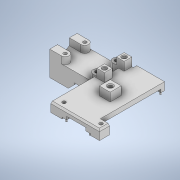
# Autodesk Inventor part: IMU_Mount
Saved by Autodesk Inventor 2022 (Build 260153000, 153)
## iProperties
Created: 2021-10-21
Part Number: IMU_Mount
Material: Generic
Document SubType Name: Modeling
Designer: kylem
Density: 1 g/cm^3
Appearance: Default
Author: kylem
Autodesk Inventor part; units mm, degrees
ref_plane "YZ Plane" through (0, 0, 0) normal (1, 0, 0) x (0, 1, 0)
ref_plane "XZ Plane" through (0, 0, 0) normal (0, 1, 0) x (-1, 0, 0)
ref_plane "XY Plane" through (0, 0, 0) normal (0, 0, 1) x (1, 0, 0)
sketch "Sketch1" plane through (0, 0, 0) normal (0, 1, 0) x (-1, 0, 0)
  point P0 (0, 0)
sketch "Sketch2" plane through (0, 0, 0) normal (0, 1, 0) x (-1, 0, 0)
  line L0 (0, 0) -> (25.5, 0)
  line L1 (25.5, 0) -> (25.5, -17.7)
  line L2 (25.5, -17.7) -> (0, -17.7)
  line L3 (0, -17.7) -> (0, 0)
  line L4 (0, 0) -> (2.5, 0)
  line L5 (2.5, 0) -> (2.5, -2.5)
  line L6 (2.5, -2.5) -> (0, -2.5)
  line L7 (0, -2.5) -> (0, 0)
  circle A0 centre (2.5, -2.5) radius 1
  line L8 (12.75, 0) -> (12.75, -1.25)
  line L9 (0, -8.85) -> (1.25, -8.85)
  circle A1 centre (2.5, -15.2) radius 1
  circle A2 centre (23, -2.5) radius 1
  circle A3 centre (23, -15.2) radius 1
  dimension "d0" = 25.5
  dimension "d1" = 17.7
  dimension "d2" = 2.5
  dimension "d3" = 2.5
  dimension "d4" = 2
  constraints: 20 end point, 4 centre point, 4 parallel, 3 horizontal, 3 symmetric about line, 2 midpoint, 2 perpendicular, 1 coincident, 1 vertical, 3 other
  measures "d0" distance of L1.end L2.end
  measures "d1" distance of L0.end L1.end
  measures "d2" distance of L5.end L6.end
  measures "d3" distance of L4.end L5.end
  measures "d4" diameter of A0
extrude "Extrusion1" add sketch "Sketch2" along normal blind 3 contours L0 L5 A0 L6 L3 | L0 L1 L2 L3 L6 A0 L5
sketch "Sketch3" plane through (0, 3, 0) normal (0, 1, 0) x (1, 0, 0)
  circle A0 centre (-2.5, 2.5) radius 1 projected
  circle A1 centre (-2.5, 2.5) radius 2.5
  circle A2 centre (-23, 2.5) radius 1 projected
  circle A3 centre (-23, 2.5) radius 2.5
  circle A4 centre (-23, 15.2) radius 1 projected
  circle A5 centre (-23, 15.2) radius 2.5
  circle A6 centre (-2.5, 15.2) radius 1 projected
  circle A7 centre (-2.5, 15.2) radius 2.5
  point P0 (0, 0)
  dimension "d7" = 5
  dimension "d8" = 5
  dimension "d9" = 5
  dimension "d10" = 5
  constraints: 4 centre point, 4 coincident
  measures "d7" diameter of A1
  measures "d8" diameter of A3
  measures "d9" diameter of A5
  measures "d10" diameter of A7
extrude "Extrusion2" add sketch "Sketch3" along normal blind 3.5
sketch "Sketch5" plane through (-2.5, 6.5, -15.2) normal (0, 1, 0) x (1, 0, 0)
  line L0 (0, 0) -> (0, 2.5)
  line L1 (2.5, 2.5) -> (-23, 2.5) projected
  line L2 (0, 2.5) -> (35, 2.5)
  line L3 (35, 2.5) -> (35, -15.2)
  line L4 (35, -15.2) -> (0, -15.2)
  line L5 (0, -15.2) -> (0, 2.5)
  circle A0 centre (0, 0) radius 1
  circle A1 centre (0, -12.7) radius 1 projected
  circle A2 centre (0, -12.7) radius 1
  point P0 (2.5, -15.2)
  point P1 (0, 1)
  point P2 (0, -1)
  point P3 (0, -11.7)
  point P4 (0, -13.7)
  dimension "d13" = 35
  constraints: 10 end point, 2 centre point, 2 coincident, 2 parallel, 1 horizontal, 1 perpendicular, 1 point on line, 1 vertical
  measures "d13" distance of L3.end L4.end
extrude "Extrusion3" add sketch "Sketch5" against normal blind 6.5 contours L0 L1 L2 L3 L4 L5 A1 A0
sketch "Sketch6" plane through (0, 6.5, 0) normal (0, 1, 0) x (1, 0, 0)
  line L0 (-2.5, 5) -> (-2.5, 12.7) projected
  line L1 (-2.5, 5) -> (1.5, 5)
  line L2 (1.5, 5) -> (1.5, 12.7)
  line L3 (1.5, 12.7) -> (-2.5, 12.7)
  line L4 (-2.5, 12.7) -> (-2.5, 5)
  point P0 (0, 0)
  dimension "d16" = 4
  constraints: 8 end point, 2 parallel, 1 horizontal, 1 perpendicular
  measures "d16" distance of L3.end L2.end
extrude "Extrusion4" cut sketch "Sketch6" against normal blind 3.5
sketch "Sketch7" plane through (0, 0, 0) normal (0, -1, 0) x (1, 0, 0)
  line L0 (0, 0) -> (4, 0)
  line L1 (-25.5, 0) -> (32.5, 0) projected
  line L2 (4, 0) -> (4, -17.7)
  line L3 (32.5, -17.7) -> (-25.5, -17.7) projected
  line L4 (4, -17.7) -> (32.5, -17.7)
  line L5 (32.5, -17.7) -> (32.5, 0)
  line L6 (32.5, 0) -> (4, 0)
  line L7 (4, 0) -> (4, -17.7)
  dimension "d19" = 4
  constraints: 12 end point, 2 parallel, 2 perpendicular, 2 point on line, 1 horizontal
  measures "d19" distance of L0.start L0.end
extrude "Extrusion5" cut sketch "Sketch7" against normal blind 3.5
sketch "Sketch9" plane through (0, 0, 0) normal (0, -1, 0) x (1, 0, 0)
  circle A0 centre (-23, -2.5) radius 1 projected
  circle A1 centre (-23, -2.5) radius 1
  circle A2 centre (-23, -15.2) radius 2.5 projected
  circle A3 centre (-23, -15.2) radius 1
  arc A4 (-23, 0) -> (-25.5, -2.5) centre (-23, -2.5) ccw projected
  line L0 (-23, 0) -> (-31, 0)
  line L1 (-31, 0) -> (-31, -17.7)
  line L2 (-31, -17.7) -> (-23, -17.7)
  line L3 (-23, -17.7) -> (-23, 0)
  circle A5 centre (-23, -15.2) radius 1
  point P0 (0, 0)
  point P1 (-23, -12.7)
  point P2 (-23, -3.5)
  point P3 (-23, -1.5)
  point P4 (-23, -14.2)
  point P5 (-23, -16.2)
  dimension "d22" = 8
  constraints: 8 end point, 3 centre point, 3 coincident, 2 parallel, 1 horizontal, 1 perpendicular
  measures "d22" distance of L2.end L1.end
extrude "Extrusion6" add sketch "Sketch9" against normal blind 6.5
sketch "Sketch12" plane through (0, 6.5, 0) normal (0, 1, 0) x (1, 0, 0)
  line L0 (-23, 17.7) -> (-31, 17.7) projected
  line L1 (-31, 17.7) -> (-26, 17.7)
  line L2 (-26, 17.7) -> (-26, 12.7)
  line L3 (-26, 12.7) -> (-31, 12.7)
  line L4 (-31, 12.7) -> (-31, 17.7)
  line L5 (-31, 17.7) -> (-31, 0) projected
  line L6 (-31, 0) -> (-26, 0)
  line L7 (-26, 0) -> (-26, 5)
  line L8 (-26, 5) -> (-31, 5)
  line L9 (-31, 5) -> (-31, 0)
  point P0 (0, 0)
  point P1 (-31, 5)
  point P2 (-26, 17.7)
  dimension "d36" = 5
  dimension "d37" = 5
  dimension "d38" = 5
  dimension "d39" = 5
  constraints: 16 end point, 4 parallel, 2 horizontal, 2 perpendicular
  measures "d36" distance of L2.end L3.end
  measures "d37" distance of L1.end L2.end
  measures "d38" distance of L8.end L7.end
  measures "d39" distance of L7.end L6.end
extrude "Extrusion9" add sketch "Sketch12" along normal blind 5.5
sketch "Sketch13" plane through (0, 12, 0) normal (0, 1, 0) x (1, 0, 0)
  line L0 (-26, 17.7) -> (-26, 12.7) projected
  line L1 (-26, 15.2) -> (-28, 15.2)
  line L2 (-31, 0) -> (-31, 17.7) projected
  circle A0 centre (-28, 15.2) radius 1.375
  line L3 (-26, 5) -> (-26, 0) projected
  line L4 (-26, 2.5) -> (-28, 2.5)
  circle A1 centre (-28, 2.5) radius 1.375
  point P0 (0, 0)
  dimension "d42" = 2
  dimension "d43" = 2.75
  dimension "d44" = 2
  dimension "d45" = 2.75
  constraints: 4 end point, 2 centre point, 2 coincident, 2 midpoint, 1 horizontal, 1 perpendicular
  measures "d42" distance of L1.start L1.end
  measures "d43" diameter of A0
  measures "d44" distance of L4.start L4.end
  measures "d45" diameter of A1
extrude "Extrusion10" cut sketch "Sketch13" against normal blind 20
sketch "Sketch14" plane through (4, 0, 0) normal (1, 0, 0) x (0, 0, -1)
  line L0 (0, 0) -> (0, 3.5) projected
  line L1 (17.7, 3.5) -> (0, 3.5) projected
  line L2 (0, 0) -> (17.7, 0)
  line L3 (17.7, 0) -> (17.7, 3.5)
  line L4 (17.7, 3.5) -> (0, 3.5)
  line L5 (0, 3.5) -> (0, 0)
  constraints: 8 end point, 2 parallel, 1 horizontal, 1 perpendicular
extrude "Extrusion11" add sketch "Sketch14" along normal blind 2
sketch "Sketch15" plane through (0, 0, 0) normal (0, -1, 0) x (1, 0, 0)
  line L0 (6, 0) -> (6, -17.7) projected
  line L1 (6, 0) -> (2.5, 0)
  line L2 (2.5, 0) -> (2.5, -2.5)
  line L3 (2.5, -2.5) -> (6, -2.5)
  line L4 (6, -2.5) -> (6, 0)
  line L5 (6, -17.7) -> (2.5, -17.7)
  line L6 (2.5, -17.7) -> (2.5, -15.2)
  line L7 (2.5, -15.2) -> (6, -15.2)
  line L8 (6, -15.2) -> (6, -17.7)
  circle A0 centre (2.5, -2.5) radius 1.375
  circle A1 centre (2.5, -15.2) radius 1.375
  point P0 (0, 0)
  dimension "d50" = 3.5
  dimension "d51" = 2.5
  dimension "d52" = 3.5
  dimension "d53" = 2.5
  dimension "d54" = 2.75
  dimension "d55" = 2.75
  constraints: 16 end point, 4 parallel, 2 centre point, 2 coincident, 2 horizontal, 2 perpendicular
  measures "d50" distance of L3.end L2.end
  measures "d51" distance of L2.end L1.end
  measures "d52" distance of L6.end L7.end
  measures "d53" distance of L5.end L6.end
  measures "d54" diameter of A0
  measures "d55" diameter of A1
extrude "Extrusion12" cut sketch "Sketch15" against normal blind 19 contours A0 L2 L3 | L3 L2 A0 | A1 L6 L7 | L7 L6 A1
sketch "Sketch16" plane through (0, 6.5, 0) normal (0, 1, 0) x (1, 0, 0)
  arc A0 (-23, 12.7) -> (-23, 17.7) centre (-23, 15.2) ccw projected
  circle A1 centre (-23, 15.2) radius 1
  arc A2 (-23, 0) -> (-23, 5) centre (-23, 2.5) ccw projected
  circle A3 centre (-23, 2.5) radius 1
  point P0 (0, 0)
  dimension "d58" = 2
  dimension "d59" = 2
  constraints: 2 centre point, 2 coincident
  measures "d58" diameter of A1
  measures "d59" diameter of A3
extrude "Extrusion13" cut sketch "Sketch16" against normal blind 19
sketch "Sketch18" plane through (0, 3.5, 0) normal (0, -1, 0) x (1, 0, 0)
  line L0 (6, 0) -> (6, -17.7) projected
  line L1 (6, 0) -> (16, 0)
  line L2 (16, 0) -> (16, -5)
  line L3 (16, -5) -> (6, -5)
  line L4 (6, -5) -> (6, 0)
  line L5 (32.5, 0) -> (32.5, -17.7) projected
  line L6 (32.5, -17.7) -> (6, -17.7)
  line L7 (6, -17.7) -> (6, 0)
  line L8 (6, 0) -> (32.5, 0)
  line L9 (32.5, 0) -> (32.5, -17.7)
  point P0 (0, 0)
  point P1 (6, -17.7)
  point P2 (6, -5)
  dimension "d66" = 10
  dimension "d67" = 5
  constraints: 16 end point, 4 parallel, 2 horizontal, 2 perpendicular
  measures "d66" distance of L2.end L3.end
  measures "d67" distance of L1.end L2.end
extrude "Extrusion15" cut sketch "Sketch18" against normal blind 19 contours L3 L2 L8 L5 L6 L0
sketch "Sketch19" plane through (0, 6.5, 0) normal (0, 1, 0) x (1, 0, 0)
  line L0 (6, 0) -> (6, 17.7) projected
  line L1 (-2.5, 0) -> (16, 0) projected
  line L2 (6, 4.9914) -> (16, 4.9914)
  line L3 (16, 4.9914) -> (16, 0)
  line L4 (16, 0) -> (6, 0)
  line L5 (6, 0) -> (6, 4.9914)
  line L6 (6, 0) -> (16, 0)
  line L7 (16, 0) -> (16, -16)
  line L8 (16, -16) -> (6, -16)
  line L9 (6, -16) -> (6, 0)
  line L10 (16, -16) -> (28.75, -16)
  line L11 (28.75, -16) -> (28.75, -24)
  line L12 (28.75, -24) -> (16, -24)
  line L13 (16, -24) -> (16, -16)
  line L14 (16, -24) -> (6, -24)
  line L15 (6, -24) -> (6, -16)
  line L16 (6, -16) -> (16, -16)
  line L17 (16, -16) -> (16, -24)
  point P0 (0, 0)
  point P1 (6, 0)
  dimension "d70" = 16
  dimension "d71" = 12.75
  dimension "d72" = 8
  constraints: 32 end point, 8 parallel, 4 horizontal, 4 perpendicular, 2 point on line
  measures "d70" distance of L6.end L7.end
  measures "d71" distance of L11.end L12.end
  measures "d72" distance of L10.end L11.end
extrude "Extrusion16" add sketch "Sketch19" against normal blind 3 contours L1 L7 L8 L9 | L8 L13 L14 L15 | L10 L11 L12 L13
sketch "Sketch20" plane through (6, 6.5, 0) normal (-1, 0, 0) x (0, 0, 1)
  line L0 (24, 0) -> (16, 0) projected
  line L1 (0, -3) -> (0, -6.5) projected
  line L2 (24, 0) -> (0, 0)
  line L3 (0, 0) -> (0, -3)
  line L4 (0, -3) -> (24, -3)
  line L5 (24, -3) -> (24, 0)
  point P0 (16, 0)
  constraints: 8 end point, 2 parallel, 1 horizontal, 1 perpendicular
extrude "Extrusion17" add sketch "Sketch20" along normal blind 7.5
sketch "Sketch21" plane through (-31, 0, -17.7) normal (-1, 0, 0) x (0, 0, 1)
  line L0 (17.7, 12) -> (12.7, 12) projected
  line L1 (0, 0) -> (17.7, 0)
  line L2 (17.7, 0) -> (17.7, 12)
  line L3 (17.7, 12) -> (0, 12)
  line L4 (0, 12) -> (0, 0)
  point P0 (17.7, 0)
  constraints: 8 end point, 2 parallel, 1 horizontal, 1 perpendicular
extrude "Extrusion18" cut sketch "Sketch21" against normal blind 1
sketch "Sketch22" plane through (0, 6.5, 0) normal (0, 1, 0) x (1, 0, 0)
  circle A0 centre (2.5, 2.5) radius 1.375 projected
  line L0 (2.5, 2.5) -> (0.5, 2.5)
  line L1 (0.5, 2.5) -> (0.5, 0)
  line L2 (0.5, 0) -> (4.5, 0)
  line L3 (4.5, 0) -> (4.5, 5)
  line L4 (4.5, 5) -> (0.5, 5)
  line L5 (0.5, 5) -> (0.5, 0)
  circle A1 centre (2.5, 15.2) radius 1.375 projected
  line L6 (2.5, 15.2) -> (0.5, 15.2)
  line L7 (0.5, 15.2) -> (0.5, 12.7)
  line L8 (0.5, 12.7) -> (2.5, 12.7)
  line L9 (2.5, 12.7) -> (2.5, 15.2)
  line L10 (0.5, 12.7) -> (4.5, 12.7)
  line L11 (4.5, 12.7) -> (4.5, 17.7)
  line L12 (4.5, 17.7) -> (0.5, 17.7)
  line L13 (0.5, 17.7) -> (0.5, 12.7)
  point P0 (0, 0)
  dimension "d79" = 2
  dimension "d80" = 2.5
  dimension "d81" = 4
  dimension "d82" = 5
  dimension "d83" = 2
  dimension "d84" = 2.5
  dimension "d85" = 4
  dimension "d86" = 5
  constraints: 28 end point, 6 parallel, 4 horizontal, 4 perpendicular
  measures "d79" distance of L0.start L0.end
  measures "d80" distance of L0.end L1.end
  measures "d81" distance of L4.end L3.end
  measures "d82" distance of L3.end L2.end
  measures "d83" distance of L8.end L7.end
  measures "d84" distance of L7.end L6.end
  measures "d85" distance of L12.end L11.end
  measures "d86" distance of L11.end L10.end
extrude "Extrusion19" add sketch "Sketch22" along normal blind 5.5 contours L5 L4 L3 L2 L1 | A1 L6 L13 L12 L11 L10 L9 | A1 L9 L8 L7 L6
sketch "Sketch23" plane through (0, 6.5, 0) normal (0, 1, 0) x (1, 0, 0)
  line L0 (28.75, -16) -> (28.75, -24) projected
  line L1 (28.75, -24) -> (-1.5, -24) projected
  line L2 (28.75, -16) -> (-1.5, -16)
  line L3 (-1.5, -16) -> (-1.5, -24)
  line L4 (-1.5, -24) -> (28.75, -24)
  line L5 (28.75, -24) -> (28.75, -16)
  point P0 (0, 0)
  constraints: 8 end point, 2 parallel, 1 horizontal, 1 perpendicular
extrude "Extrusion20" add sketch "Sketch23" along normal blind 5.5
sketch "Sketch24" plane through (0, 0, 0) normal (0, -1, 0) x (1, 0, 0)
  line L0 (6, -17.7) -> (-30, -17.7) projected
  line L1 (6, -17.7) -> (7.5, -17.7)
  line L2 (7.5, -17.7) -> (7.5, -7.7)
  line L3 (7.5, -7.7) -> (6, -7.7)
  line L4 (6, -7.7) -> (6, -17.7)
  point P0 (0, 0)
  dimension "d91" = 1.5
  dimension "d92" = 10
  constraints: 8 end point, 2 parallel, 1 horizontal, 1 perpendicular
  measures "d91" distance of L3.end L2.end
  measures "d92" distance of L2.end L1.end
extrude "Extrusion21" add sketch "Sketch24" against normal blind 6.5
sketch "Sketch25" plane through (0, 3.5, 0) normal (0, -1, 0) x (1, 0, 0)
  line L0 (16, 16) -> (16, -5) projected
  line L1 (-1.5, 16) -> (16, 16) projected
  line L2 (16, 16) -> (-1.5, 16)
  line L3 (6, 0) -> (6, -5) projected
  line L4 (-1.5, 16) -> (-1.5, 0) projected
  line L5 (6, 0) -> (-1.5, 0)
  line L6 (-1.5, 0) -> (-1.5, 16)
  line L7 (-1.5, 16) -> (6, 16)
  line L8 (6, 16) -> (6, 0)
  point P0 (0, 0)
  constraints: 10 end point, 2 horizontal, 2 parallel, 1 perpendicular
extrude "Extrusion22" add sketch "Sketch25" along normal blind 3.5
sketch "Sketch26" plane through (0, 6.5, 0) normal (0, 1, 0) x (1, 0, 0)
  line L0 (7.5, 17.7) -> (7.5, 7.7) projected
  line L1 (6, 5) -> (6, 7.7) projected
  line L2 (7.5, 7.7) -> (6, 7.7)
  line L3 (6, 7.7) -> (6, 5)
  line L4 (6, 5) -> (7.5, 5)
  line L5 (7.5, 5) -> (7.5, 7.7)
  point P0 (0, 0)
  constraints: 8 end point, 2 parallel, 1 horizontal, 1 perpendicular
extrude "Extrusion23" add sketch "Sketch26" against normal blind 3
sketch "Sketch29" plane through (-1.5, 3.5, 24) normal (0, 0, 1) x (1, 0, 0)
  line L0 (0, 0) -> (0, 8.5) projected
  line L1 (30.25, 8.5) -> (0, 8.5) projected
  line L2 (0, 0) -> (30.25, 0)
  line L3 (30.25, 0) -> (30.25, 8.5)
  line L4 (30.25, 8.5) -> (0, 8.5)
  line L5 (0, 8.5) -> (0, 0)
  point P0 (1.5, -3.5)
  constraints: 8 end point, 2 parallel, 1 horizontal, 1 perpendicular
extrude "Extrusion27" cut sketch "Sketch29" against normal blind 2.2
sketch "Sketch30" plane through (-1.5, 3.5, 16) normal (0, 0, 1) x (1, 0, 0)
  line L0 (30.25, 0) -> (0, 0) projected
  line L1 (0, 0) -> (7.5, 0)
  line L2 (7.5, 0) -> (7.5, -3.5)
  line L3 (7.5, -3.5) -> (0, -3.5)
  line L4 (0, -3.5) -> (0, 0)
  point P0 (1.5, -3.5)
  constraints: 8 end point, 2 parallel, 1 horizontal, 1 perpendicular
extrude "Extrusion28" cut sketch "Sketch30" against normal blind 2
sketch "Sketch31" plane through (28.75, 3.5, 16) normal (0, 0, -1) x (-1, 0, 0)
  line L0 (0, 0) -> (0, 8.5) projected
  line L1 (12.75, 3) -> (12.75, 0) projected
  line L2 (0, 8.5) -> (12.75, 8.5)
  line L3 (12.75, 8.5) -> (12.75, 0)
  line L4 (12.75, 0) -> (0, 0)
  line L5 (0, 0) -> (0, 8.5)
  line L6 (30.25, 3) -> (30.25, 8.5) projected
  line L7 (30.25, 3) -> (12.75, 3)
  line L8 (12.75, 3) -> (12.75, 8.5)
  line L9 (12.75, 8.5) -> (30.25, 8.5)
  line L10 (30.25, 8.5) -> (30.25, 3)
  point P0 (28.75, -3.5)
  constraints: 16 end point, 4 parallel, 2 horizontal, 2 perpendicular
extrude "Extrusion29" add sketch "Sketch31" along normal blind 2
sketch "Sketch35" plane through (16, 3.5, -5) normal (1, 0, 0) x (0, 0, -1)
  line L0 (-19, 3) -> (0, 3) projected
  line L1 (2.7, 0) -> (0, 0) projected
  line L2 (-19, 3) -> (0, 3)
  line L3 (0, 3) -> (0, 0)
  line L4 (0, 0) -> (-19, 0)
  line L5 (-19, 0) -> (-19, 3)
  point P0 (-5, -3.5)
  constraints: 8 end point, 2 parallel, 1 horizontal, 1 perpendicular
extrude "Extrusion32" cut sketch "Sketch35" against normal blind 4
sketch "Sketch36" plane through (0, 6.5, 0) normal (0, 1, 0) x (1, 0, 0)
  circle A0 centre (-2.5, 2.5) radius 1 projected
  arc A1 (-2.5, 5) -> (-2.5, 0) centre (-2.5, 2.5) ccw projected
  arc A2 (-2.5, 5) -> (-2.5, 0) centre (-2.5, 2.5) ccw
  line L0 (0.5, 0) -> (-5.8371, 0)
  line L1 (-5.8371, 0) -> (-5.8371, 5)
  line L2 (-5.8371, 5) -> (0.5, 5)
  line L3 (0.5, 5) -> (0.5, 0)
  line L4 (0.5, 17.7) -> (0.5, 12.7) projected
  line L5 (0.5, 12.7) -> (-2.5, 12.7)
  line L6 (-2.5, 17.7) -> (0.5, 17.7)
  line L7 (0.5, 17.7) -> (0.5, 12.7)
  arc A3 (-2.5, 17.7) -> (-2.5, 12.7) centre (-2.5, 15.2) ccw projected
  arc A4 (-2.5, 17.7) -> (-2.5, 12.7) centre (-2.5, 15.2) ccw
  circle A5 centre (-2.5, 2.5) radius 1
  circle A6 centre (-2.5, 15.2) radius 1
  circle A7 centre (-23, 15.2) radius 1 projected
  circle A8 centre (-23, 15.2) radius 1
  circle A9 centre (-23, 2.5) radius 1 projected
  circle A10 centre (-23, 2.5) radius 1
  arc A11 (-23, 0) -> (-23, 5) centre (-23, 2.5) ccw
  line L8 (-23, 5) -> (-23, 12.7) projected
  arc A12 (-23, 12.7) -> (-23, 17.7) centre (-23, 15.2) ccw
  line L9 (-26, 17.7) -> (-26, 12.7) projected
  line L10 (-23, 0) -> (-2.5, 0) projected
  line L11 (-26, 17.7) -> (-23, 17.7)
  line L12 (-23, 0) -> (-26, 0)
  line L13 (-30, 5) -> (-26, 5)
  line L14 (-26, 12.7) -> (-30, 12.7)
  line L15 (-30, 12.7) -> (-30, 5)
  line L16 (-26, 0) -> (-26, 5)
  line L17 (-26, 12.7) -> (-26, 17.7)
  line L18 (-23, 3.5) -> (-23, 1.5)
  line L19 (-23, 16.2) -> (-23, 14.2)
  line L20 (-23, 12.7) -> (-23, 5)
  point P0 (0, 0)
  constraints: 34 end point, 16 point on circle, 11 parallel, 8 centre point, 8 coincident, 4 horizontal, 4 perpendicular, 4 point on line, 1 concentric
extrude "Extrusion33" add sketch "Sketch36" along normal blind 1 contours L2 L3 L0 A1 | L4 L5 A3 L6 | L12 L16 L13 L15 L14 L9 L11 A12 L8 A11
sketch "Sketch37" plane through (0, 0, 0) normal (0, -1, 0) x (1, 0, 0)
  line L0 (7.5, -5) -> (7.5, -17.7) projected
  line L1 (-30, 0) -> (-30, -17.7) projected
  line L2 (7.5, -17.7) -> (-30, -17.7)
  line L3 (-30, -17.7) -> (-30, 0)
  line L4 (7.5, 0) -> (7.5, -17.7)
  line L5 (-1.5, 14) -> (-1.5, 0) projected
  line L6 (7.5, -17.7) -> (4.5, -17.7) projected
  line L7 (-1.5, 14) -> (6, 14)
  line L8 (6, 14) -> (6, 0)
  line L9 (6, -17.7) -> (-1.5, -17.7)
  line L10 (-1.5, 0) -> (-1.5, 14)
  line L11 (-30, 0) -> (-1.5, 0)
  line L12 (6, 0) -> (7.5, 0)
  circle A0 centre (-28, -2.5) radius 1.375 projected
  circle A1 centre (-28, -2.5) radius 1.25
  circle A2 centre (-23, -2.5) radius 1 projected
  circle A3 centre (-23, -2.5) radius 1
  circle A4 centre (-23, -15.2) radius 1 projected
  circle A5 centre (-23, -15.2) radius 1
  circle A6 centre (-28, -15.2) radius 1.375 projected
  circle A7 centre (-28, -15.2) radius 1.25
  circle A8 centre (-2.5, -15.2) radius 1 projected
  circle A9 centre (-2.5, -15.2) radius 1
  circle A10 centre (2.5, -15.2) radius 1.375 projected
  circle A11 centre (2.5, -15.2) radius 1.25
  circle A12 centre (2.5, -2.5) radius 1.375 projected
  circle A13 centre (2.5, -2.5) radius 1.25
  line L13 (7.5, -7.7) -> (6, -7.7) projected
  line L14 (6, -7.7) -> (7.5, -7.7)
  line L15 (7.5, -7.7) -> (7.5, 0)
  line L16 (7.5, 0) -> (6, 0)
  line L17 (6, 0) -> (6, -7.7)
  point P0 (0, 0)
  constraints: 26 end point, 7 centre point, 7 coincident, 7 parallel, 3 horizontal, 3 perpendicular, 1 midpoint
extrude "Extrusion34" add sketch "Sketch37" along normal blind 3.5 contours L0 L2 L1 L11 L5 L7 L8 L17 L13
chamfer "Chamfer2" distance 4 angle 45 1 edges at (28.75, 7.75, 14)
chamfer "Chamfer4" distance 0.25 angle 60 1 edges at (1.125, 12, -2.5) measured on face at (1.025, 12, -2.5)
chamfer "Chamfer5" distance 0.25 angle 60 1 edges at (1.125, 12, -15.2) measured on face at (1.025, 12, -15.2)
chamfer "Chamfer6" distance 0.25 angle 60 1 edges at (-29.375, 12, -2.5) measured on face at (-29.475, 12, -2.5)
chamfer "Chamfer7" distance 0.25 angle 60 1 edges at (-29.375, 12, -15.2) measured on face at (-29.475, 12, -15.2)
sketch "Sketch39" plane through (0, 7.5, 0) normal (0, 1, 0) x (1, 0, 0)
  circle A0 centre (-2.5, 2.5) radius 1 projected
  circle A1 centre (-2.5, 2.5) radius 1
  point P0 (0, 0)
  constraints: 1 centre point, 1 coincident
extrude "Extrusion37" cut sketch "Sketch39" against normal blind 40
sketch "Sketch41" plane through (0, 7.5, 0) normal (0, 1, 0) x (1, 0, 0)
  circle A0 centre (-2.5, 2.5) radius 1 projected
  circle A1 centre (-2.5, 2.5) radius 1.1
  circle A2 centre (-2.5, 15.2) radius 1 projected
  circle A3 centre (-2.5, 15.2) radius 1.1
  circle A4 centre (-23, 15.2) radius 1 projected
  circle A5 centre (-23, 15.2) radius 1.1
  circle A6 centre (-23, 2.5) radius 1.1
  point P0 (0, 0)
  dimension "d162" = 2.2
  dimension "d163" = 2.2
  dimension "d164" = 2.2
  dimension "d165" = 2.2
  constraints: 4 centre point, 3 coincident
  measures "d162" diameter of A1
  measures "d163" diameter of A3
  measures "d164" diameter of A5
  measures "d165" diameter of A6
extrude "Extrusion38" cut sketch "Sketch41" against normal blind 100 contours A0 | A1 | A2 | A3 | A4 | A5 | A6
sketch "Sketch43" plane through (0, 12, 0) normal (0, 1, 0) x (1, 0, 0)
  line L0 (19, -7) -> (19, -14) projected
  line L1 (19, -7) -> (15.5, -7)
  line L2 (15.5, -7) -> (15.5, -10.5)
  line L3 (15.5, -10.5) -> (19, -10.5)
  line L4 (19, -10.5) -> (19, -7)
  circle A0 centre (15.5, -10.5) radius 1.4
  point P0 (0, 0)
  dimension "d172" = 3.5
  dimension "d173" = 3.5
  dimension "d174" = 2.8
  constraints: 8 end point, 2 parallel, 1 centre point, 1 coincident, 1 horizontal, 1 perpendicular
  measures "d172" distance of L3.end L2.end
  measures "d173" distance of L2.end L1.end
  measures "d174" diameter of A0
extrude "Extrusion40" cut sketch "Sketch43" against normal blind 8.5 contours A0 L2 L3 | L3 L2 A0
sketch "Sketch44" plane through (-30, 0, -17.7) normal (-1, 0, 0) x (0, 0, 1)
  line L0 (17.7, 7.5) -> (17.7, 12) projected
  line L1 (5, 7.5) -> (0, 7.5) projected
  line L2 (17.7, 12) -> (0, 12)
  line L3 (0, 12) -> (0, 7.5)
  line L4 (0, 7.5) -> (17.7, 7.5)
  line L5 (17.7, 7.5) -> (17.7, 12)
  point P0 (17.7, 0)
  constraints: 8 end point, 2 parallel, 1 horizontal, 1 perpendicular
extrude "Extrusion41" cut sketch "Sketch44" against normal blind 10
sketch "Sketch45" plane through (0, 7.5, 0) normal (0, 1, 0) x (1, 0, 0)
  line L0 (-30, 17.7) -> (-23, 17.7) projected
  line L1 (-30, 0) -> (-25.7284, 0)
  line L2 (-25.7284, 0) -> (-25.7284, 17.7)
  line L3 (-25.7284, 17.7) -> (-30, 17.7)
  line L4 (-30, 17.7) -> (-30, 0)
  point P0 (0, 0)
  constraints: 8 end point, 2 parallel, 1 horizontal, 1 perpendicular, 1 point on line
extrude "Extrusion42" add sketch "Sketch45" against normal blind 11
sketch "Sketch47" plane through (-30, 0, -17.7) normal (-1, 0, 0) x (0, 0, 1)
  line L0 (17.7, -3.5) -> (17.7, 6.5) projected
  line L1 (5, 7.5) -> (0, 7.5) projected
  line L2 (17.7, -3.5) -> (0, -3.5)
  line L3 (0, -3.5) -> (0, 7.5)
  line L4 (0, 7.5) -> (17.7, 7.5)
  line L5 (17.7, 7.5) -> (17.7, -3.5)
  circle A0 centre (8.85, 0) radius 1.4 projected
  circle A1 centre (8.85, 0) radius 1.4
  point P0 (17.7, 0)
  constraints: 8 end point, 2 parallel, 1 centre point, 1 coincident, 1 horizontal, 1 perpendicular
extrude "Extrusion44" add sketch "Sketch47" along normal blind 0.5
sketch "Sketch51" plane through (0, 12, 0) normal (0, 1, 0) x (1, 0, 0)
  line L0 (0.5, 5) -> (0.5, 0) projected
  line L1 (1.5, 5) -> (-2.5, 5) projected
  line L2 (0.5, 0) -> (0, 0)
  line L3 (0, 0) -> (0, 5)
  line L4 (0, 5) -> (0.5, 5)
  line L5 (0.5, 5) -> (0.5, 0)
  line L6 (4.5, 0) -> (5, 0)
  line L7 (5, 0) -> (5, 5)
  line L8 (5, 5) -> (4.5, 5)
  line L9 (4.5, 5) -> (4.5, 0)
  line L10 (0.5, 17.7) -> (0.5, 12.7) projected
  line L11 (7.5, 17.7) -> (-30.5, 17.7) projected
  line L12 (0.5, 12.7) -> (0, 12.7)
  line L13 (0, 12.7) -> (0, 17.7)
  line L14 (0, 17.7) -> (0.5, 17.7)
  line L15 (0.5, 17.7) -> (0.5, 12.7)
  line L16 (4.5, 17.7) -> (4.5, 12.7) projected
  line L17 (4.5, 12.7) -> (5, 12.7)
  line L18 (5, 12.7) -> (5, 17.7)
  line L19 (5, 17.7) -> (4.5, 17.7)
  line L20 (4.5, 17.7) -> (4.5, 12.7)
  dimension "d208" = 0.5
  dimension "d209" = 5
  constraints: 32 end point, 8 parallel, 5 point on line, 4 horizontal, 4 perpendicular
  measures "d208" distance of L8.end L7.end
  measures "d209" distance of L7.end L6.end
extrude "Extrusion46" add sketch "Sketch51" against normal blind 8.5
sketch "Sketch53" plane through (0, -3.5, 0) normal (0, -1, 0) x (1, 0, 0)
  line L0 (-30.5, -17.7) -> (-30.5, 0) projected
  line L1 (7.5, -17.7) -> (-30.5, -17.7) projected
  line L2 (-30.5, 0) -> (-14.5, 0)
  line L3 (-14.5, 0) -> (-14.5, -17.7)
  line L4 (-14.5, -17.7) -> (-30.5, -17.7)
  line L5 (-30.5, -17.7) -> (-30.5, 0)
  arc A0 (-23, -5) -> (-23, 0) centre (-23, -2.5) ccw projected
  circle A1 centre (-23, -2.5) radius 1.1
  circle A2 centre (-23, -15.2) radius 1.1 projected
  circle A3 centre (-23, -15.2) radius 1.1
  point P0 (0, 0)
  point P1 (-30.5, -4.2879)
  dimension "d221" = 16
  constraints: 8 end point, 2 centre point, 2 coincident, 2 parallel, 1 horizontal, 1 perpendicular, 1 point on line
  measures "d221" distance of L3.end L4.end
extrude "Extrusion48" add sketch "Sketch53" along normal blind 5
sketch "Sketch54" plane through (-30.5, 0, -17.7) normal (-1, 0, 0) x (0, 0, 1)
  line L0 (0, -8.5) -> (17.7, -8.5) projected
  line L1 (0, -8.5) -> (8.85, -8.5)
  line L2 (8.85, -8.5) -> (8.85, -2.75)
  circle A0 centre (8.85, -2.75) radius 4.75
  point P0 (17.7, 0)
  point P1 (12.0613, -8.5)
  point P2 (5.6387, -8.5)
  dimension "d224" = 5.75
  dimension "d229" = 9.5
  constraints: 4 end point, 1 centre point, 1 coincident, 1 midpoint, 1 perpendicular
  measures "d224" distance of L1.end L2.end
  measures "d229" diameter of A0
sketch "Sketch55" plane through (-30, 0, -8.85) normal (-1, 0, 0) x (0, 0, 1)
  circle A0 centre (0, 0) radius 1.4
  point P0 (8.85, 0)
  constraints: 1 centre point
extrude "Extrusion49" add sketch "Sketch55" along normal blind 0.5
sketch "Sketch56" plane through (-23, 3, -5) normal (1, 0, 0) x (0, 0, -1)
  line L0 (0, 0) -> (0, 4.5) projected
  line L1 (7.7, 4.5) -> (7.7, 0) projected
  line L2 (0, 0) -> (7.7, 0)
  line L3 (7.7, 0) -> (7.7, 4.5)
  line L4 (7.7, 4.5) -> (0, 4.5)
  line L5 (0, 4.5) -> (0, 0)
  point P0 (-5, -3)
  constraints: 8 end point, 2 parallel, 1 horizontal, 1 perpendicular
extrude "Extrusion50" cut sketch "Sketch56" against normal blind 10
extrude "Extrusion51" cut sketch "Sketch54" against normal blind 5.5
sketch "Sketch57" plane through (-25, 0, -17.7) normal (-1, 0, 0) x (0, 0, 1)
  circle A0 centre (8.85, -2.75) radius 4.75 projected
  circle A1 centre (8.85, -2.75) radius 1.4
  point P0 (17.7, 0)
  point P1 (5.6387, -8.5)
  point P2 (12.0613, -8.5)
  dimension "d232" = 2.8
  constraints: 1 centre point, 1 coincident, 1 other
  measures "d232" diameter of A1
extrude "Extrusion52" cut sketch "Sketch57" against normal blind 10 contours A1
chamfer "Chamfer13" distance 4 angle 45 1 edges at (-14.5, -8.5, -8.85)
chamfer "Chamfer14" distance 2 angle 45 1 edges at (-30.5, -2.75, -13.6)
sketch "Sketch58" plane through (0, 12, 0) normal (0, 1, 0) x (1, 0, 0)
  line L0 (6, -14) -> (-1.5, -14) projected
  line L1 (0, -14) -> (17.75, -14)
  line L2 (17.75, -14) -> (17.75, -2) projected
  line L3 (17.75, -14) -> (10.75, -14)
  line L4 (10.75, -14) -> (10.75, -2)
  line L5 (10.75, -2) -> (17.75, -2)
  line L6 (17.75, -2) -> (17.75, -14)
  line L7 (10.75, -2) -> (14.286, -2)
  line L8 (14.286, -2) -> (14.286, -5.536)
  line L9 (14.286, -5.536) -> (10.75, -5.536)
  line L10 (10.75, -5.536) -> (10.75, -2)
  circle A0 centre (14.286, -5.536) radius 1.4
  point P0 (0, 0)
  dimension "d241" = 17.75
  dimension "d242" = 7
  dimension "d243" = 12
  dimension "d244" = 3.536
  dimension "d245" = 3.536
  dimension "d246" = 2.8
  constraints: 18 end point, 4 parallel, 2 horizontal, 2 perpendicular, 1 centre point, 1 coincident, 1 collinear, 1 point on line
  measures "d241" distance of L1.start L1.end
  measures "d242" distance of L4.end L5.end
  measures "d243" distance of L3.end L4.end
  measures "d244" distance of L8.end L9.end
  measures "d245" distance of L7.end L8.end
  measures "d246" diameter of A0
extrude "Extrusion53" add sketch "Sketch58" against normal blind 8.5 contours L4 L9 A0 L8 L5 L2 L1 | L4 L5 L8 A0 L9
chamfer "Chamfer16" distance 0.5 angle 45 1 edges at (12.886, 12, 5.536)
sketch "Sketch59" plane through (0, 12, 0) normal (0, 1, 0) x (1, 0, 0)
  line L0 (17.75, -14) -> (24.75, -14) projected
  line L1 (24.75, -14) -> (28.75, -18) projected
  line L2 (17.75, -14) -> (26.75, -14)
  line L3 (26.75, -14) -> (26.75, -16)
  line L4 (26.75, -16) -> (17.75, -16)
  line L5 (17.75, -16) -> (17.75, -14)
  point P0 (0, 0)
  constraints: 8 end point, 2 parallel, 1 horizontal, 1 midpoint, 1 perpendicular
extrude "Extrusion54" cut sketch "Sketch59" against normal blind 8.5 contours L0 L1 L4 L5
sketch "Sketch60" plane through (-1.5, 6.5, 0) normal (-1, 0, 0) x (0, 0, 1)
  line L0 (2, 2) -> (2, 0) projected
  line L1 (2, 0) -> (5.56, 0)
  line L2 (14, 0) -> (0, 0) projected
  line L3 (5.56, 0) -> (9.12, 0)
  line L4 (21.8, 5.5) -> (21.8, -3) projected
  line L5 (9.12, 0) -> (21.8, 0)
  line L6 (21.8, 0) -> (21.8, 5.5)
  line L7 (21.8, 5.5) -> (9.12, 5.5)
  line L8 (9.12, 5.5) -> (9.12, 0)
  point P0 (0, -6.5)
  dimension "d257" = 3.56
  dimension "d258" = 3.56
  constraints: 12 end point, 2 parallel, 2 point on line, 1 horizontal, 1 perpendicular
  measures "d257" distance of L0.end L1.end
  measures "d258" distance of L1.end L3.end
extrude "Extrusion55" cut sketch "Sketch60" against normal blind 50
sketch "Sketch61" plane through (0, -3.5, 0) normal (0, -1, 0) x (1, 0, 0)
  line L0 (12, -5) -> (7.5, -5) projected
  line L1 (6, -7.7) -> (6, 14) projected
  line L2 (7.5, -5) -> (6, -5)
  line L3 (6, -5) -> (6, -7.7)
  line L4 (6, -7.7) -> (7.5, -7.7)
  line L5 (7.5, -7.7) -> (7.5, -5)
  line L6 (7.5, -5) -> (7.5, -17.7) projected
  line L7 (6, -7.7) -> (7.5, -7.7)
  line L8 (7.5, -7.7) -> (7.5, -17.7)
  line L9 (7.5, -17.7) -> (6, -17.7)
  line L10 (6, -17.7) -> (6, -7.7)
  point P0 (0, 0)
  constraints: 16 end point, 4 parallel, 2 horizontal, 2 perpendicular
extrude "Extrusion56" cut sketch "Sketch61" against normal blind 50
sketch "Sketch62" plane through (0, 3.5, 0) normal (0, -1, 0) x (1, 0, 0)
  line L0 (28.75, 21.8) -> (-1.5, 21.8) projected
  line L1 (28.75, 21.8) -> (24, 21.8)
  line L2 (24, 21.8) -> (24, 14.0848)
  line L3 (24, 14.0848) -> (28.75, 14.0848)
  line L4 (28.75, 14.0848) -> (28.75, 21.8)
  point P0 (0, 0)
  dimension "d263" = 4.75
  constraints: 8 end point, 2 parallel, 1 horizontal, 1 perpendicular
  measures "d263" distance of L3.end L2.end
extrude "Extrusion57" cut sketch "Sketch62" against normal blind 50
sketch "Sketch63" plane through (0, 6.5, 0) normal (0, 1, 0) x (1, 0, 0)
  line L0 (6, 5) -> (6, 17.7) projected
  line L1 (6, 17.7) -> (-14.5, 17.7) projected
  line L2 (6, 5) -> (6, 17.7)
  line L3 (6, 17.7) -> (6, 19.92)
  line L4 (6, 19.92) -> (37.2084, 19.92)
  line L5 (17.75, -16) -> (24, -16) projected
  line L6 (24, -16) -> (24, 25.1533)
  line L7 (6, 5) -> (12, 5) projected
  line L8 (6, 5) -> (12, 5)
  line L9 (12, -2) -> (12, 5) projected
  line L10 (12, 5) -> (12, -2)
  line L11 (17.75, -2) -> (10.75, -2) projected
  line L12 (12, -2) -> (17.75, -2)
  line L13 (17.75, -2) -> (17.75, -16)
  line L14 (17.75, -9.12) -> (17.75, -2) projected
  point P0 (0, 0)
  point P1 (24, 19.92)
  dimension "d266" = 2.22
  constraints: 16 end point, 4 collinear, 2 perpendicular, 1 point on line, 1 vertical
  measures "d266" distance of L0.end L3.end
extrude "Extrusion58" add sketch "Sketch63" against normal blind 3
sketch "Sketch64" plane through (0, 6.5, 0) normal (0, 1, 0) x (1, 0, 0)
  line L0 (24, -21.8) -> (-1.5, -21.8) projected
  line L1 (24, -21.8) -> (-1.5, -21.8)
  line L2 (-1.5, -21.8) -> (-1.5, -28.28)
  line L3 (-1.5, -28.28) -> (24, -28.28)
  line L4 (24, -28.28) -> (24, -21.8)
  point P0 (0, 0)
  dimension "d269" = 6.48
  constraints: 8 end point, 2 parallel, 1 horizontal, 1 perpendicular
  measures "d269" distance of L2.end L1.end
extrude "Extrusion59" add sketch "Sketch64" against normal blind 3
sketch "Sketch66" plane through (0, 3.5, 0) normal (0, -1, 0) x (1, 0, 0)
  line L0 (6, -17.7) -> (6, -19.92) projected
  line L1 (6, -19.92) -> (8.76, -19.92)
  line L2 (8.76, -19.92) -> (8.76, -17.44)
  line L3 (8.76, -17.44) -> (6, -17.44)
  line L4 (6, -17.44) -> (6, -19.92)
  line L5 (6, -19.92) -> (24, -19.92) projected
  line L6 (24, -19.92) -> (26.48, -19.92)
  line L7 (26.48, -19.92) -> (26.48, -17.44)
  line L8 (26.48, -17.44) -> (24, -17.44)
  line L9 (24, -17.44) -> (24, -19.92)
  line L10 (-1.5, 28.28) -> (24, 28.28) projected
  line L11 (24, 28.28) -> (21.24, 28.28)
  line L12 (21.24, 28.28) -> (21.24, 25.8)
  line L13 (21.24, 25.8) -> (24, 25.8)
  line L14 (24, 25.8) -> (24, 28.28)
  line L15 (6, -17.7) -> (6, 14) projected
  line L16 (6, 14) -> (6, 29.3242)
  line L17 (6, 28.28) -> (8.76, 28.28)
  line L18 (8.76, 28.28) -> (8.76, 25.8)
  line L19 (8.76, 25.8) -> (6, 25.8)
  line L20 (6, 25.8) -> (6, 28.28)
  line L21 (24, -19.92) -> (21.24, -19.92)
  line L22 (21.24, -19.92) -> (21.24, -17.44)
  line L23 (21.24, -17.44) -> (24, -17.44)
  line L24 (24, -17.44) -> (24, -19.92)
  point P0 (0, 0)
  dimension "d272" = 2.76
  dimension "d273" = 2.48
  dimension "d274" = 2.48
  dimension "d275" = 2.48
  dimension "d276" = 2.76
  dimension "d277" = 2.48
  dimension "d278" = 2.76
  dimension "d279" = 2.48
  dimension "d280" = 2.76
  dimension "d281" = 2.48
  constraints: 42 end point, 10 parallel, 5 horizontal, 5 perpendicular, 2 point on line, 1 vertical
  measures "d272" distance of L3.end L2.end
  measures "d273" distance of L2.end L1.end
  measures "d274" distance of L8.end L7.end
  measures "d275" distance of L7.end L6.end
  measures "d276" distance of L13.end L12.end
  measures "d277" distance of L12.end L11.end
  measures "d278" distance of L18.end L19.end
  measures "d279" distance of L17.end L18.end
  measures "d280" distance of L22.end L23.end
  measures "d281" distance of L21.end L22.end
extrude "Extrusion60" add sketch "Sketch66" along normal blind 2 contours L4 L3 L2 L1 L0 | L22 L23 L9 L5 | L10 L18 L19 L16 | L10 L14 L13 L12
sketch "Sketch67" plane through (0, 1.5, 0) normal (0, -1, 0) x (1, 0, 0)
  line L0 (8.76, 25.8) -> (8.76, 28.28) projected
  line L1 (8.76, 27.04) -> (7.38, 27.04)
  line L2 (6, 28.28) -> (6, 25.8) projected
  line L3 (21.24, 28.28) -> (21.24, 25.8) projected
  line L4 (21.24, 27.04) -> (22.62, 27.04)
  line L5 (24, -17.44) -> (21.24, -17.44) projected
  line L6 (22.62, -17.44) -> (22.62, -18.68)
  line L7 (8.76, -19.92) -> (8.76, -17.44) projected
  line L8 (8.76, -18.68) -> (7.38, -18.68)
  circle A0 centre (7.38, 27.04) radius 0.5
  circle A1 centre (22.62, 27.04) radius 0.5
  circle A2 centre (22.62, -18.68) radius 0.5
  circle A3 centre (7.38, -18.68) radius 0.5
  point P0 (0, 0)
  dimension "d284" = 1.38
  dimension "d285" = 1.38
  dimension "d286" = 1.24
  dimension "d287" = 1.38
  dimension "d288" = 1
  dimension "d289" = 1
  dimension "d290" = 1
  dimension "d291" = 1
  constraints: 8 end point, 4 centre point, 4 coincident, 4 midpoint, 2 horizontal, 1 perpendicular, 1 vertical
  measures "d284" distance of L1.start L1.end
  measures "d285" distance of L4.start L4.end
  measures "d286" distance of L6.start L6.end
  measures "d287" distance of L8.start L8.end
  measures "d288" diameter of A0
  measures "d289" diameter of A1
  measures "d290" diameter of A2
  measures "d291" diameter of A3
extrude "Extrusion61" add sketch "Sketch67" along normal blind 3
sketch "Sketch69" plane through (0, 6.5, 0) normal (0, 1, 0) x (1, 0, 0)
  line L0 (-1.5, -28.28) -> (-1.5, 0) projected
  line L1 (-1.5, -28.28) -> (6, -28.28)
  line L2 (6, -28.28) -> (6, -21.78)
  line L3 (6, -21.78) -> (-1.5, -21.78)
  line L4 (-1.5, -21.78) -> (-1.5, -28.28)
  line L5 (-1.5, -28.28) -> (24, -28.28) projected
  line L6 (24, -28.28) -> (30, -28.28)
  line L7 (30, -28.28) -> (30, -21.78)
  line L8 (30, -21.78) -> (24, -21.78)
  line L9 (24, 17.44) -> (24, -25.8) projected
  line L10 (24, -28.28) -> (24, 19.92) projected
  line L11 (24, -28.28) -> (24, -21.78)
  point P0 (0, 0)
  dimension "d294" = 7.5
  dimension "d295" = 6.5
  dimension "d296" = 6
  dimension "d297" = 6.5
  constraints: 16 end point, 3 perpendicular, 2 horizontal, 2 parallel, 1 collinear, 1 point on line
  measures "d294" distance of L3.end L2.end
  measures "d295" distance of L2.end L1.end
  measures "d296" distance of L5.end L6.end
  measures "d297" distance of L6.end L7.end
extrude "Extrusion62" add sketch "Sketch69" against normal blind 6
sketch "Sketch70" plane through (6, 0.5, 21.78) normal (1, 0, 0) x (0, 0, -1)
  line L0 (-6.5, 1) -> (-6.5, 0) projected
  line L1 (-6.5, 1) -> (-6.5, 0)
  line L2 (0, 0) -> (-6.5, 0) projected
  line L3 (-6.5, 0) -> (0, 0)
  line L4 (0, 3) -> (0, 0) projected
  line L5 (0, 0) -> (0, 3)
  line L6 (-4.02, 3) -> (0, 3) projected
  line L7 (0, 3) -> (-4.02, 3)
  line L8 (-4.02, 3) -> (-4.02, 1)
  line L9 (-6.5, 1) -> (-4.02, 1) projected
  line L10 (-4.02, 1) -> (-6.5, 1)
  point P0 (21.78, -0.5)
  constraints: 12 end point, 5 collinear, 1 perpendicular
extrude "Extrusion63" cut sketch "Sketch70" against normal blind 0.25
sketch "Sketch71" plane through (24, 0.5, 21.78) normal (-1, 0, 0) x (0, 0, 1)
  line L0 (0, 3) -> (4.02, 3) projected
  line L1 (4.02, 3) -> (0, 3)
  line L2 (0, 3) -> (0, 0) projected
  line L3 (0, 3) -> (0, 0)
  line L4 (6.5, 0) -> (0, 0) projected
  line L5 (0, 0) -> (6.5, 0)
  line L6 (6.5, 1) -> (6.5, 0) projected
  line L7 (6.5, 0) -> (6.5, 1)
  line L8 (4.02, 1) -> (6.5, 1) projected
  line L9 (6.5, 1) -> (4.02, 1)
  line L10 (4.02, 1) -> (4.02, 3)
  point P0 (-21.78, -0.5)
  constraints: 12 end point, 4 collinear, 2 perpendicular
extrude "Extrusion64" cut sketch "Sketch71" against normal blind 0.25
sketch "Sketch72" plane through (0, 0.5, 0) normal (0, -1, 0) x (1, 0, 0)
  line L0 (5.75, 25.8) -> (5.75, 21.78) projected
  line L1 (5.75, 21.78) -> (3, 21.78)
  line L2 (3, 21.78) -> (3, 24.28)
  line L3 (3, 24.28) -> (5.75, 24.28)
  line L4 (5.75, 24.28) -> (5.75, 21.78)
  line L5 (24.25, 21.78) -> (30, 21.78) projected
  line L6 (24.25, 21.78) -> (27, 21.78)
  line L7 (27, 21.78) -> (27, 24.28)
  line L8 (27, 24.28) -> (24.25, 24.28)
  line L9 (24.25, 24.28) -> (24.25, 21.78)
  circle A0 centre (3, 24.28) radius 1.1
  circle A1 centre (27, 24.28) radius 1.1
  point P0 (0, 0)
  dimension "d304" = 2.75
  dimension "d305" = 2.5
  dimension "d306" = 2.75
  dimension "d307" = 2.5
  dimension "d308" = 2.2
  dimension "d309" = 2.2
  constraints: 16 end point, 4 parallel, 2 centre point, 2 coincident, 2 horizontal, 2 perpendicular
  measures "d304" distance of L2.end L3.end
  measures "d305" distance of L1.end L2.end
  measures "d306" distance of L8.end L7.end
  measures "d307" distance of L7.end L6.end
  measures "d308" diameter of A0
  measures "d309" diameter of A1
extrude "Extrusion65" cut sketch "Sketch72" against normal blind 9 contours A0 L2 L3 | L3 L2 A0 | A1 L8 L7 | L7 L8 A1
sketch "Sketch73" plane through (7.38, -1.5, -18.68) normal (0, -1, 0) x (1, 0, 0)
  line L0 (-0.99, 0.9698) -> (17.0121, 0.9698)
  line L1 (17.0121, 0.9698) -> (17.0121, -1.2241)
  line L2 (17.0121, -1.2241) -> (-0.99, -1.2241)
  line L3 (-0.99, -1.2241) -> (-0.99, 0.9698)
  point P0 (-7.38, 18.68)
  constraints: 8 end point, 2 parallel, 1 horizontal, 1 perpendicular
extrude "Extrusion66" cut sketch "Sketch73" against normal blind 1
chamfer "Chamfer17" distance 1 angle 45 1 edges at (14.25, 6.5, 28.28)
chamfer "Chamfer18" distance 1 angle 45 1 edges at (30, 6.5, 24.53)
sketch "Sketch74" plane through (7.38, -1.5, 27.04) normal (0, -1, 0) x (1, 0, 0)
  line L0 (-1.1159, 0.8172) -> (16.0517, 0.8172)
  line L1 (16.0517, 0.8172) -> (16.0517, -0.9359)
  line L2 (16.0517, -0.9359) -> (-1.1159, -0.9359)
  line L3 (-1.1159, -0.9359) -> (-1.1159, 0.8172)
  point P0 (-7.38, -27.04)
  constraints: 8 end point, 2 parallel, 1 horizontal, 1 perpendicular
extrude "Extrusion67" cut sketch "Sketch74" against normal blind 1
body "Solid1"
